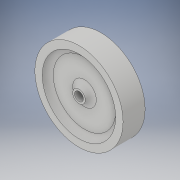
# Autodesk Inventor part: Part7
Saved by Autodesk Inventor 2018 (Build 220112000, 112)
## iProperties
Created: 2018-07-02
Part Number: Part7
Material: Generic
Document SubType Name: Modeling
Designer: s-2512711
Density: 1 g/cm^3
Appearance: Default
Author: s-2512711
Autodesk Inventor part; units mm, degrees
ref_plane "YZ Plane" through (0, 0, 0) normal (1, 0, 0) x (0, 1, 0)
ref_plane "XZ Plane" through (0, 0, 0) normal (0, 1, 0) x (-1, 0, 0)
ref_plane "XY Plane" through (0, 0, 0) normal (0, 0, 1) x (1, 0, 0)
sketch "Sketch1" plane through (0, 0, 0) normal (0, 0, 1) x (1, 0, 0)
  circle A0 centre (0, 0) radius 7.6581
  circle A1 centre (0, 0) radius 10.1981
  circle A2 centre (0, 0) radius 76.2
  circle A3 centre (0, 0) radius 63.5
  dimension "d0" = 15.3162
  dimension "d1" = 20.3962
  dimension "d2" = 152.4
  dimension "d3" = 127
  constraints: 4 centre point, 4 coincident
  measures "d0" diameter of A0
  measures "d1" diameter of A1
  measures "d2" diameter of A2
  measures "d3" diameter of A3
extrude "Extrusion1" add sketch "Sketch1" along normal blind 38.1
sketch "Sketch2" plane through (0, 0, 38.1) normal (0, 0, 1) x (1, 0, 0)
  circle A0 centre (0, 0) radius 10.1981
  circle A1 centre (0, 0) radius 63.5
  constraints: 2 centre point, 2 coincident
extrude "Extrusion2" add sketch "Sketch2" against normal blind 28.575
sketch "Sketch3" plane through (0, 0, 38.1) normal (0, 0, 1) x (1, 0, 0)
  circle A0 centre (0, 0) radius 10.8988
  circle A1 centre (0, 0) radius 63.5
  constraints: 2 centre point, 2 coincident
extrude "Extrusion3" cut sketch "Sketch3" against normal blind 9.525
fillet "Fillet1" radius 9.525 2 edges at (-10.1981, 0, 9.525) (-63.5, 0, 9.525)
fillet "Fillet2" radius 9.525 2 edges at (-63.5, 0, 28.575) (-10.8988, 0, 28.575)
sketch "Sketch4" plane through (0, 0, 0) normal (0, 0, -1) x (-1, 0, 0)
  line L0 (-9.1597, 73.9585) -> (12.5018, 73.9585) construction
  line L1 (12.5018, 73.9585) -> (12.5018, 68.6979) construction
  line L2 (12.5018, 68.6979) -> (-9.1597, 68.6979) construction
  line L3 (-9.1597, 68.6979) -> (-9.1597, 73.9585) construction
  spline S0 degree 2 poles (-6.9244, 72.9038) (-6.9244, 72.7062) (-7.0651, 72.3506) (-7.1911, 72.227) knots 0 0 0 1 2 2 2
  spline S1 degree 2 poles (-7.1911, 72.227) (-7.3492, 72.0714) (-7.7765, 71.9109) (-8.1026, 71.9109) knots 0 0 0 1 2 2 2
  line L4 (-8.1026, 71.9109) -> (-8.4459, 71.9109)
  line L5 (-8.4459, 71.9109) -> (-8.4459, 70.7747)
  line L6 (-8.4459, 70.7747) -> (-8.851, 70.7747)
  line L7 (-8.851, 70.7747) -> (-8.851, 73.8227)
  line L8 (-8.851, 73.8227) -> (-8.0853, 73.8227)
  spline S2 degree 2 poles (-8.0853, 73.8227) (-7.8136, 73.8227) (-7.4332, 73.7338) (-7.2874, 73.6325) knots 0 0 0 1 2 2 2
  spline S3 degree 2 poles (-7.2874, 73.6325) (-7.117, 73.5164) (-6.9244, 73.1582) (-6.9244, 72.9038) knots 0 0 0 1 2 2 2
  spline S4 degree 2 poles (-7.3467, 72.8915) (-7.3467, 73.0496) (-7.4554, 73.2817) (-7.5666, 73.3558) knots 0 0 0 1 2 2 2
  spline S5 degree 2 poles (-7.5666, 73.3558) (-7.6629, 73.4201) (-7.9198, 73.4719) (-8.11, 73.4719) knots 0 0 0 1 2 2 2
  line L9 (-8.11, 73.4719) -> (-8.4459, 73.4719)
  line L10 (-8.4459, 73.4719) -> (-8.4459, 72.2567)
  line L11 (-8.4459, 72.2567) -> (-8.1692, 72.2567)
  spline S6 degree 2 poles (-8.1692, 72.2567) (-7.9222, 72.2567) (-7.6184, 72.3357) (-7.5196, 72.4395) knots 0 0 0 1 2 2 2
  spline S7 degree 2 poles (-7.5196, 72.4395) (-7.4282, 72.5309) (-7.3467, 72.7458) (-7.3467, 72.8915) knots 0 0 0 1 2 2 2
  line L12 (-5.3559, 72.6494) -> (-5.3757, 72.6494)
  spline S8 degree 2 poles (-5.3757, 72.6494) (-5.4201, 72.6618) (-5.5164, 72.6667) (-5.5831, 72.6667) knots 0 0 0 1 2 2 2
  spline S9 degree 2 poles (-5.5831, 72.6667) (-5.7387, 72.6667) (-6.045, 72.5309) (-6.1833, 72.3975) knots 0 0 0 1 2 2 2
  line L13 (-6.1833, 72.3975) -> (-6.1833, 70.7747)
  line L14 (-6.1833, 70.7747) -> (-6.5687, 70.7747)
  line L15 (-6.5687, 70.7747) -> (-6.5687, 73.0619)
  line L16 (-6.5687, 73.0619) -> (-6.1833, 73.0619)
  line L17 (-6.1833, 73.0619) -> (-6.1833, 72.7211)
  spline S10 degree 2 poles (-6.1833, 72.7211) (-5.9734, 72.9088) (-5.6597, 73.0619) (-5.5115, 73.0619) knots 0 0 0 1 2 2 2
  spline S11 degree 2 poles (-5.5115, 73.0619) (-5.4522, 73.0619) (-5.3929, 73.057) (-5.3559, 73.0496) knots 0 0 0 1 2 2 2
  line L18 (-5.3559, 73.0496) -> (-5.3559, 72.6494)
  spline S12 degree 2 poles (-4.0641, 70.7228) (-4.6124, 70.7228) (-5.2151, 71.3378) (-5.2151, 71.9059) knots 0 0 0 1 2 2 2
  spline S13 degree 2 poles (-5.2151, 71.9059) (-5.2151, 72.4642) (-4.6297, 73.1261) (-4.1579, 73.1261) knots 0 0 0 1 2 2 2
  spline S14 degree 2 poles (-4.1579, 73.1261) (-3.9455, 73.1261) (-3.617, 73.0026) (-3.496, 72.8717) knots 0 0 0 1 2 2 2
  spline S15 degree 2 poles (-3.496, 72.8717) (-3.3725, 72.7408) (-3.2416, 72.3629) (-3.2416, 72.0887) knots 0 0 0 1 2 2 2
  line L19 (-3.2416, 72.0887) -> (-3.2416, 71.8788)
  line L20 (-3.2416, 71.8788) -> (-4.8248, 71.8788)
  spline S16 degree 2 poles (-4.8248, 71.8788) (-4.8248, 71.4811) (-4.4247, 71.0587) (-4.069, 71.0587) knots 0 0 0 1 2 2 2
  spline S17 degree 2 poles (-4.069, 71.0587) (-3.943, 71.0587) (-3.6985, 71.1155) (-3.5997, 71.16) knots 0 0 0 1 2 2 2
  spline S18 degree 2 poles (-3.5997, 71.16) (-3.496, 71.2094) (-3.3527, 71.2959) (-3.3058, 71.3354) knots 0 0 0 1 2 2 2
  line L21 (-3.3058, 71.3354) -> (-3.2835, 71.3354)
  line L22 (-3.2835, 71.3354) -> (-3.2835, 70.9155)
  spline S19 degree 2 poles (-3.2835, 70.9155) (-3.3502, 70.8883) (-3.5528, 70.8093) (-3.6318, 70.787) knots 0 0 0 1 2 2 2
  spline S20 degree 2 poles (-3.6318, 70.787) (-3.743, 70.7549) (-3.9258, 70.7228) (-4.0641, 70.7228) knots 0 0 0 1 2 2 2
  spline S21 degree 2 poles (-3.617, 72.1727) (-3.6219, 72.3283) (-3.6862, 72.5556) (-3.7479, 72.6321) knots 0 0 0 1 2 2 2
  spline S22 degree 2 poles (-3.7479, 72.6321) (-3.8146, 72.7186) (-4.0246, 72.81) (-4.1802, 72.81) knots 0 0 0 1 2 2 2
  spline S23 degree 2 poles (-4.1802, 72.81) (-4.3333, 72.81) (-4.5482, 72.7186) (-4.6371, 72.6297) knots 0 0 0 1 2 2 2
  spline S24 degree 2 poles (-4.6371, 72.6297) (-4.7236, 72.5383) (-4.8125, 72.3184) (-4.8248, 72.1727) knots 0 0 0 1 2 2 2
  line L23 (-4.8248, 72.1727) -> (-3.617, 72.1727)
  spline S25 degree 2 poles (-2.1597, 70.7302) (-2.4734, 70.7302) (-2.8266, 71.0884) (-2.8266, 71.4762) knots 0 0 0 1 2 2 2
  line L24 (-2.8266, 71.4762) -> (-2.8266, 72.7433)
  line L25 (-2.8266, 72.7433) -> (-3.0859, 72.7433)
  line L26 (-3.0859, 72.7433) -> (-3.0859, 73.0619)
  line L27 (-3.0859, 73.0619) -> (-2.8266, 73.0619)
  line L28 (-2.8266, 73.0619) -> (-2.8266, 73.7189)
  line L29 (-2.8266, 73.7189) -> (-2.4413, 73.7189)
  line L30 (-2.4413, 73.7189) -> (-2.4413, 73.0619)
  line L31 (-2.4413, 73.0619) -> (-1.7324, 73.0619)
  line L32 (-1.7324, 73.0619) -> (-1.7324, 72.7433)
  line L33 (-1.7324, 72.7433) -> (-2.4413, 72.7433)
  line L34 (-2.4413, 72.7433) -> (-2.4413, 71.654)
  spline S26 degree 2 poles (-2.4413, 71.654) (-2.4413, 71.4811) (-2.4289, 71.2909) (-2.3869, 71.2094) knots 0 0 0 1 2 2 2
  spline S27 degree 2 poles (-2.3869, 71.2094) (-2.3524, 71.1378) (-2.1967, 71.0661) (-2.0634, 71.0661) knots 0 0 0 1 2 2 2
  spline S28 degree 2 poles (-2.0634, 71.0661) (-1.9695, 71.0661) (-1.7941, 71.123) (-1.7546, 71.1402) knots 0 0 0 1 2 2 2
  line L35 (-1.7546, 71.1402) -> (-1.7324, 71.1402)
  line L36 (-1.7324, 71.1402) -> (-1.7324, 70.7944)
  spline S29 degree 2 poles (-1.7324, 70.7944) (-1.8411, 70.7648) (-2.0634, 70.7302) (-2.1597, 70.7302) knots 0 0 0 1 2 2 2
  spline S30 degree 2 poles (-0.4554, 70.7228) (-1.0037, 70.7228) (-1.6064, 71.3378) (-1.6064, 71.9059) knots 0 0 0 1 2 2 2
  spline S31 degree 2 poles (-1.6064, 71.9059) (-1.6064, 72.4642) (-1.021, 73.1261) (-0.5492, 73.1261) knots 0 0 0 1 2 2 2
  spline S32 degree 2 poles (-0.5492, 73.1261) (-0.3368, 73.1261) (-0.0083, 73.0026) (0.1127, 72.8717) knots 0 0 0 1 2 2 2
  spline S33 degree 2 poles (0.1127, 72.8717) (0.2362, 72.7408) (0.3671, 72.3629) (0.3671, 72.0887) knots 0 0 0 1 2 2 2
  line L37 (0.3671, 72.0887) -> (0.3671, 71.8788)
  line L38 (0.3671, 71.8788) -> (-1.2161, 71.8788)
  spline S34 degree 2 poles (-1.2161, 71.8788) (-1.2161, 71.4811) (-0.816, 71.0587) (-0.4603, 71.0587) knots 0 0 0 1 2 2 2
  spline S35 degree 2 poles (-0.4603, 71.0587) (-0.3344, 71.0587) (-0.0898, 71.1155) (0.009, 71.16) knots 0 0 0 1 2 2 2
  spline S36 degree 2 poles (0.009, 71.16) (0.1127, 71.2094) (0.256, 71.2959) (0.3029, 71.3354) knots 0 0 0 1 2 2 2
  line L39 (0.3029, 71.3354) -> (0.3251, 71.3354)
  line L40 (0.3251, 71.3354) -> (0.3251, 70.9155)
  spline S37 degree 2 poles (0.3251, 70.9155) (0.2585, 70.8883) (0.0559, 70.8093) (-0.0231, 70.787) knots 0 0 0 1 2 2 2
  spline S38 degree 2 poles (-0.0231, 70.787) (-0.1343, 70.7549) (-0.3171, 70.7228) (-0.4554, 70.7228) knots 0 0 0 1 2 2 2
  spline S39 degree 2 poles (-0.0083, 72.1727) (-0.0132, 72.3283) (-0.0775, 72.5556) (-0.1392, 72.6321) knots 0 0 0 1 2 2 2
  spline S40 degree 2 poles (-0.1392, 72.6321) (-0.2059, 72.7186) (-0.4159, 72.81) (-0.5715, 72.81) knots 0 0 0 1 2 2 2
  spline S41 degree 2 poles (-0.5715, 72.81) (-0.7246, 72.81) (-0.9395, 72.7186) (-1.0284, 72.6297) knots 0 0 0 1 2 2 2
  spline S42 degree 2 poles (-1.0284, 72.6297) (-1.1149, 72.5383) (-1.2038, 72.3184) (-1.2161, 72.1727) knots 0 0 0 1 2 2 2
  line L41 (-1.2161, 72.1727) -> (-0.0083, 72.1727)
  line L42 (2.5531, 70.7747) -> (2.1678, 70.7747)
  line L43 (2.1678, 70.7747) -> (2.1678, 72.0788)
  spline S43 degree 2 poles (2.1678, 72.0788) (2.1678, 72.2369) (2.1381, 72.5086) (2.0937, 72.5901) knots 0 0 0 1 2 2 2
  spline S44 degree 2 poles (2.0937, 72.5901) (2.0467, 72.6766) (1.8788, 72.7606) (1.7355, 72.7606) knots 0 0 0 1 2 2 2
  spline S45 degree 2 poles (1.7355, 72.7606) (1.5923, 72.7606) (1.2885, 72.6074) (1.1427, 72.4839) knots 0 0 0 1 2 2 2
  line L44 (1.1427, 72.4839) -> (1.1427, 70.7747)
  line L45 (1.1427, 70.7747) -> (0.7574, 70.7747)
  line L46 (0.7574, 70.7747) -> (0.7574, 73.0619)
  line L47 (0.7574, 73.0619) -> (1.1427, 73.0619)
  line L48 (1.1427, 73.0619) -> (1.1427, 72.8075)
  spline S46 degree 2 poles (1.1427, 72.8075) (1.3156, 72.9631) (1.6491, 73.1261) (1.8368, 73.1261) knots 0 0 0 1 2 2 2
  spline S47 degree 2 poles (1.8368, 73.1261) (2.1727, 73.1261) (2.5531, 72.6815) (2.5531, 72.2592) knots 0 0 0 1 2 2 2
  line L49 (2.5531, 72.2592) -> (2.5531, 70.7747)
  line L50 (4.8527, 70.7747) -> (4.4674, 70.7747)
  line L51 (4.4674, 70.7747) -> (4.4674, 71.0069)
  spline S48 degree 2 poles (4.4674, 71.0069) (4.3784, 70.9328) (4.2475, 70.834) (4.1586, 70.792) knots 0 0 0 1 2 2 2
  spline S49 degree 2 poles (4.1586, 70.792) (4.0771, 70.7525) (3.9017, 70.7105) (3.7856, 70.7105) knots 0 0 0 1 2 2 2
  spline S50 degree 2 poles (3.7856, 70.7105) (3.5979, 70.7105) (3.2818, 70.8661) (3.1706, 71.0167) knots 0 0 0 1 2 2 2
  spline S51 degree 2 poles (3.1706, 71.0167) (3.0595, 71.1674) (2.936, 71.612) (2.936, 71.901) knots 0 0 0 1 2 2 2
  spline S52 degree 2 poles (2.936, 71.901) (2.936, 72.2023) (3.0916, 72.642) (3.2274, 72.8075) knots 0 0 0 1 2 2 2
  spline S53 degree 2 poles (3.2274, 72.8075) (3.3534, 72.9557) (3.7066, 73.1261) (3.9017, 73.1261) knots 0 0 0 1 2 2 2
  spline S54 degree 2 poles (3.9017, 73.1261) (4.0722, 73.1261) (4.3266, 73.0496) (4.4674, 72.9705) knots 0 0 0 1 2 2 2
  line L52 (4.4674, 72.9705) -> (4.4674, 73.9585)
  line L53 (4.4674, 73.9585) -> (4.8527, 73.9585)
  line L54 (4.8527, 73.9585) -> (4.8527, 70.7747)
  line L55 (4.4674, 71.3304) -> (4.4674, 72.6519)
  spline S55 degree 2 poles (4.4674, 72.6519) (4.3241, 72.7211) (4.0969, 72.7729) (3.9659, 72.7729) knots 0 0 0 1 2 2 2
  spline S56 degree 2 poles (3.9659, 72.7729) (3.6695, 72.7729) (3.3336, 72.3283) (3.3336, 71.9084) knots 0 0 0 1 2 2 2
  spline S57 degree 2 poles (3.3336, 71.9084) (3.3336, 71.5033) (3.5905, 71.076) (3.8746, 71.076) knots 0 0 0 1 2 2 2
  spline S58 degree 2 poles (3.8746, 71.076) (4.0252, 71.076) (4.3315, 71.2143) (4.4674, 71.3304) knots 0 0 0 1 2 2 2
  spline S59 degree 2 poles (7.4116, 70.7302) (7.0979, 70.7302) (6.7447, 71.0884) (6.7447, 71.4762) knots 0 0 0 1 2 2 2
  line L56 (6.7447, 71.4762) -> (6.7447, 72.7433)
  line L57 (6.7447, 72.7433) -> (6.4854, 72.7433)
  line L58 (6.4854, 72.7433) -> (6.4854, 73.0619)
  line L59 (6.4854, 73.0619) -> (6.7447, 73.0619)
  line L60 (6.7447, 73.0619) -> (6.7447, 73.7189)
  line L61 (6.7447, 73.7189) -> (7.13, 73.7189)
  line L62 (7.13, 73.7189) -> (7.13, 73.0619)
  line L63 (7.13, 73.0619) -> (7.8389, 73.0619)
  line L64 (7.8389, 73.0619) -> (7.8389, 72.7433)
  line L65 (7.8389, 72.7433) -> (7.13, 72.7433)
  line L66 (7.13, 72.7433) -> (7.13, 71.654)
  spline S60 degree 2 poles (7.13, 71.654) (7.13, 71.4811) (7.1424, 71.2909) (7.1844, 71.2094) knots 0 0 0 1 2 2 2
  spline S61 degree 2 poles (7.1844, 71.2094) (7.219, 71.1378) (7.3746, 71.0661) (7.508, 71.0661) knots 0 0 0 1 2 2 2
  spline S62 degree 2 poles (7.508, 71.0661) (7.6018, 71.0661) (7.7772, 71.123) (7.8167, 71.1402) knots 0 0 0 1 2 2 2
  line L67 (7.8167, 71.1402) -> (7.8389, 71.1402)
  line L68 (7.8389, 71.1402) -> (7.8389, 70.7944)
  spline S63 degree 2 poles (7.8389, 70.7944) (7.7303, 70.7648) (7.508, 70.7302) (7.4116, 70.7302) knots 0 0 0 1 2 2 2
  line L69 (9.9187, 70.7747) -> (9.5334, 70.7747)
  line L70 (9.5334, 70.7747) -> (9.5334, 72.0788)
  spline S64 degree 2 poles (9.5334, 72.0788) (9.5334, 72.2369) (9.5037, 72.5086) (9.4593, 72.5901) knots 0 0 0 1 2 2 2
  spline S65 degree 2 poles (9.4593, 72.5901) (9.4123, 72.6766) (9.2444, 72.7606) (9.1011, 72.7606) knots 0 0 0 1 2 2 2
  spline S66 degree 2 poles (9.1011, 72.7606) (8.9579, 72.7606) (8.654, 72.6074) (8.5083, 72.4839) knots 0 0 0 1 2 2 2
  line L71 (8.5083, 72.4839) -> (8.5083, 70.7747)
  line L72 (8.5083, 70.7747) -> (8.123, 70.7747)
  line L73 (8.123, 70.7747) -> (8.123, 73.9585)
  line L74 (8.123, 73.9585) -> (8.5083, 73.9585)
  line L75 (8.5083, 73.9585) -> (8.5083, 72.8075)
  spline S67 degree 2 poles (8.5083, 72.8075) (8.6812, 72.9631) (9.0147, 73.1261) (9.2024, 73.1261) knots 0 0 0 1 2 2 2
  spline S68 degree 2 poles (9.2024, 73.1261) (9.5383, 73.1261) (9.9187, 72.6815) (9.9187, 72.2592) knots 0 0 0 1 2 2 2
  line L76 (9.9187, 72.2592) -> (9.9187, 70.7747)
  line L77 (10.8524, 70.7747) -> (10.467, 70.7747)
  line L78 (10.467, 70.7747) -> (10.467, 73.0619)
  line L79 (10.467, 73.0619) -> (10.8524, 73.0619)
  line L80 (10.8524, 73.0619) -> (10.8524, 70.7747)
  line L81 (10.8795, 73.4423) -> (10.4423, 73.4423)
  line L82 (10.4423, 73.4423) -> (10.4423, 73.8424)
  line L83 (10.4423, 73.8424) -> (10.8795, 73.8424)
  line L84 (10.8795, 73.8424) -> (10.8795, 73.4423)
  spline S69 degree 2 poles (12.0355, 70.7203) (11.8058, 70.7203) (11.4081, 70.8438) (11.2772, 70.913) knots 0 0 0 1 2 2 2
  line L85 (11.2772, 70.913) -> (11.2772, 71.3453)
  line L86 (11.2772, 71.3453) -> (11.297, 71.3453)
  spline S70 degree 2 poles (11.297, 71.3453) (11.3464, 71.3057) (11.4797, 71.2119) (11.5909, 71.16) knots 0 0 0 1 2 2 2
  spline S71 degree 2 poles (11.5909, 71.16) (11.6872, 71.1131) (11.9243, 71.0439) (12.0503, 71.0439) knots 0 0 0 1 2 2 2
  spline S72 degree 2 poles (12.0503, 71.0439) (12.1417, 71.0439) (12.3517, 71.0859) (12.4011, 71.1205) knots 0 0 0 1 2 2 2
  spline S73 degree 2 poles (12.4011, 71.1205) (12.4727, 71.1674) (12.5369, 71.2736) (12.5369, 71.3823) knots 0 0 0 1 2 2 2
  spline S74 degree 2 poles (12.5369, 71.3823) (12.5369, 71.5182) (12.3887, 71.6589) (12.1985, 71.7059) knots 0 0 0 1 2 2 2
  spline S75 degree 2 poles (12.1985, 71.7059) (12.1244, 71.7232) (11.8873, 71.7726) (11.786, 71.7997) knots 0 0 0 1 2 2 2
  spline S76 degree 2 poles (11.786, 71.7997) (11.5242, 71.8763) (11.2871, 72.1925) (11.2871, 72.4172) knots 0 0 0 1 2 2 2
  spline S77 degree 2 poles (11.2871, 72.4172) (11.2871, 72.7285) (11.7539, 73.1163) (12.1392, 73.1163) knots 0 0 0 1 2 2 2
  spline S78 degree 2 poles (12.1392, 73.1163) (12.3294, 73.1163) (12.7147, 73.0224) (12.8457, 72.9508) knots 0 0 0 1 2 2 2
  line L87 (12.8457, 72.9508) -> (12.8457, 72.5383)
  line L88 (12.8457, 72.5383) -> (12.8259, 72.5383)
  spline S79 degree 2 poles (12.8259, 72.5383) (12.6777, 72.6568) (12.3171, 72.7927) (12.1318, 72.7927) knots 0 0 0 1 2 2 2
  spline S80 degree 2 poles (12.1318, 72.7927) (11.9416, 72.7927) (11.6798, 72.6321) (11.6798, 72.4716) knots 0 0 0 1 2 2 2
  spline S81 degree 2 poles (11.6798, 72.4716) (11.6798, 72.3259) (11.8354, 72.1851) (12.0083, 72.1406) knots 0 0 0 1 2 2 2
  spline S82 degree 2 poles (12.0083, 72.1406) (12.0923, 72.1184) (12.3047, 72.0739) (12.4208, 72.0467) knots 0 0 0 1 2 2 2
  spline S83 degree 2 poles (12.4208, 72.0467) (12.6728, 71.9825) (12.9296, 71.6886) (12.9296, 71.4342) knots 0 0 0 1 2 2 2
  spline S84 degree 2 poles (12.9296, 71.4342) (12.9296, 71.286) (12.8135, 71.0242) (12.6999, 70.9278) knots 0 0 0 1 2 2 2
  spline S85 degree 2 poles (12.6999, 70.9278) (12.5789, 70.8266) (12.2701, 70.7203) (12.0355, 70.7203) knots 0 0 0 1 2 2 2
  line L89 (-8.4879, 65.7562) -> (-8.8732, 65.7562)
  line L90 (-8.8732, 65.7562) -> (-8.8732, 68.0435)
  line L91 (-8.8732, 68.0435) -> (-8.4879, 68.0435)
  line L92 (-8.4879, 68.0435) -> (-8.4879, 65.7562)
  line L93 (-8.4607, 68.4238) -> (-8.8979, 68.4238)
  line L94 (-8.8979, 68.4238) -> (-8.8979, 68.824)
  line L95 (-8.8979, 68.824) -> (-8.4607, 68.824)
  line L96 (-8.4607, 68.824) -> (-8.4607, 68.4238)
  spline S86 degree 2 poles (-7.3047, 65.7019) (-7.5344, 65.7019) (-7.9321, 65.8254) (-8.063, 65.8945) knots 0 0 0 1 2 2 2
  line L97 (-8.063, 65.8945) -> (-8.063, 66.3268)
  line L98 (-8.063, 66.3268) -> (-8.0433, 66.3268)
  spline S87 degree 2 poles (-8.0433, 66.3268) (-7.9939, 66.2873) (-7.8605, 66.1934) (-7.7493, 66.1416) knots 0 0 0 1 2 2 2
  spline S88 degree 2 poles (-7.7493, 66.1416) (-7.653, 66.0946) (-7.4159, 66.0255) (-7.2899, 66.0255) knots 0 0 0 1 2 2 2
  spline S89 degree 2 poles (-7.2899, 66.0255) (-7.1985, 66.0255) (-6.9886, 66.0675) (-6.9392, 66.102) knots 0 0 0 1 2 2 2
  spline S90 degree 2 poles (-6.9392, 66.102) (-6.8675, 66.149) (-6.8033, 66.2552) (-6.8033, 66.3639) knots 0 0 0 1 2 2 2
  spline S91 degree 2 poles (-6.8033, 66.3639) (-6.8033, 66.4997) (-6.9515, 66.6405) (-7.1417, 66.6874) knots 0 0 0 1 2 2 2
  spline S92 degree 2 poles (-7.1417, 66.6874) (-7.2158, 66.7047) (-7.4529, 66.7541) (-7.5542, 66.7813) knots 0 0 0 1 2 2 2
  spline S93 degree 2 poles (-7.5542, 66.7813) (-7.816, 66.8579) (-8.0532, 67.174) (-8.0532, 67.3988) knots 0 0 0 1 2 2 2
  spline S94 degree 2 poles (-8.0532, 67.3988) (-8.0532, 67.71) (-7.5863, 68.0978) (-7.201, 68.0978) knots 0 0 0 1 2 2 2
  spline S95 degree 2 poles (-7.201, 68.0978) (-7.0108, 68.0978) (-6.6255, 68.0039) (-6.4946, 67.9323) knots 0 0 0 1 2 2 2
  line L99 (-6.4946, 67.9323) -> (-6.4946, 67.5198)
  line L100 (-6.4946, 67.5198) -> (-6.5143, 67.5198)
  spline S96 degree 2 poles (-6.5143, 67.5198) (-6.6625, 67.6384) (-7.0232, 67.7742) (-7.2084, 67.7742) knots 0 0 0 1 2 2 2
  spline S97 degree 2 poles (-7.2084, 67.7742) (-7.3986, 67.7742) (-7.6604, 67.6137) (-7.6604, 67.4531) knots 0 0 0 1 2 2 2
  spline S98 degree 2 poles (-7.6604, 67.4531) (-7.6604, 67.3074) (-7.5048, 67.1666) (-7.3319, 67.1221) knots 0 0 0 1 2 2 2
  spline S99 degree 2 poles (-7.3319, 67.1221) (-7.2479, 67.0999) (-7.0355, 67.0555) (-6.9194, 67.0283) knots 0 0 0 1 2 2 2
  spline S100 degree 2 poles (-6.9194, 67.0283) (-6.6675, 66.9641) (-6.4106, 66.6701) (-6.4106, 66.4157) knots 0 0 0 1 2 2 2
  spline S101 degree 2 poles (-6.4106, 66.4157) (-6.4106, 66.2675) (-6.5267, 66.0057) (-6.6403, 65.9094) knots 0 0 0 1 2 2 2
  spline S102 degree 2 poles (-6.6403, 65.9094) (-6.7613, 65.8081) (-7.0701, 65.7019) (-7.3047, 65.7019) knots 0 0 0 1 2 2 2
  spline S103 degree 2 poles (-3.8344, 65.7044) (-4.0715, 65.7044) (-4.4642, 65.8501) (-4.605, 65.9983) knots 0 0 0 1 2 2 2
  spline S104 degree 2 poles (-4.605, 65.9983) (-4.7458, 66.144) (-4.9014, 66.5936) (-4.9014, 66.8949) knots 0 0 0 1 2 2 2
  spline S105 degree 2 poles (-4.9014, 66.8949) (-4.9014, 67.1962) (-4.7409, 67.6359) (-4.605, 67.7841) knots 0 0 0 1 2 2 2
  spline S106 degree 2 poles (-4.605, 67.7841) (-4.4692, 67.9348) (-4.0665, 68.0953) (-3.8344, 68.0953) knots 0 0 0 1 2 2 2
  spline S107 degree 2 poles (-3.8344, 68.0953) (-3.6466, 68.0953) (-3.2959, 67.9891) (-3.16, 67.92) knots 0 0 0 1 2 2 2
  line L101 (-3.16, 67.92) -> (-3.16, 67.4877)
  line L102 (-3.16, 67.4877) -> (-3.1823, 67.4877)
  spline S108 degree 2 poles (-3.1823, 67.4877) (-3.2243, 67.5223) (-3.3527, 67.6112) (-3.4441, 67.6581) knots 0 0 0 1 2 2 2
  spline S109 degree 2 poles (-3.4441, 67.6581) (-3.5256, 67.6977) (-3.743, 67.7594) (-3.8418, 67.7594) knots 0 0 0 1 2 2 2
  spline S110 degree 2 poles (-3.8418, 67.7594) (-4.1406, 67.7594) (-4.5037, 67.3074) (-4.5037, 66.8949) knots 0 0 0 1 2 2 2
  spline S111 degree 2 poles (-4.5037, 66.8949) (-4.5037, 66.4923) (-4.153, 66.0403) (-3.8418, 66.0403) knots 0 0 0 1 2 2 2
  spline S112 degree 2 poles (-3.8418, 66.0403) (-3.6541, 66.0403) (-3.3132, 66.1959) (-3.1823, 66.3169) knots 0 0 0 1 2 2 2
  line L103 (-3.1823, 66.3169) -> (-3.16, 66.3169)
  line L104 (-3.16, 66.3169) -> (-3.16, 65.8847)
  spline S113 degree 2 poles (-3.16, 65.8847) (-3.2169, 65.8575) (-3.3898, 65.7809) (-3.4589, 65.7636) knots 0 0 0 1 2 2 2
  spline S114 degree 2 poles (-3.4589, 65.7636) (-3.5577, 65.734) (-3.7133, 65.7044) (-3.8344, 65.7044) knots 0 0 0 1 2 2 2
  spline S115 degree 2 poles (-0.9296, 66.8998) (-0.9296, 66.3219) (-1.4854, 65.692) (-1.9497, 65.692) knots 0 0 0 1 2 2 2
  spline S116 degree 2 poles (-1.9497, 65.692) (-2.4265, 65.692) (-2.9723, 66.3416) (-2.9723, 66.8998) knots 0 0 0 1 2 2 2
  spline S117 degree 2 poles (-2.9723, 66.8998) (-2.9723, 67.4729) (-2.4092, 68.1077) (-1.9497, 68.1077) knots 0 0 0 1 2 2 2
  spline S118 degree 2 poles (-1.9497, 68.1077) (-1.4854, 68.1077) (-0.9296, 67.4754) (-0.9296, 66.8998) knots 0 0 0 1 2 2 2
  spline S119 degree 2 poles (-1.3273, 66.8998) (-1.3273, 67.3444) (-1.6509, 67.7767) (-1.9497, 67.7767) knots 0 0 0 1 2 2 2
  spline S120 degree 2 poles (-1.9497, 67.7767) (-2.2486, 67.7767) (-2.5747, 67.3444) (-2.5747, 66.8998) knots 0 0 0 1 2 2 2
  spline S121 degree 2 poles (-2.5747, 66.8998) (-2.5747, 66.4676) (-2.2486, 66.023) (-1.9497, 66.023) knots 0 0 0 1 2 2 2
  spline S122 degree 2 poles (-1.9497, 66.023) (-1.6533, 66.023) (-1.3273, 66.4602) (-1.3273, 66.8998) knots 0 0 0 1 2 2 2
  line L105 (-0.1417, 65.7562) -> (-0.527, 65.7562)
  line L106 (-0.527, 65.7562) -> (-0.527, 68.9401)
  line L107 (-0.527, 68.9401) -> (-0.1417, 68.9401)
  line L108 (-0.1417, 68.9401) -> (-0.1417, 65.7562)
  spline S123 degree 2 poles (1.0414, 65.7019) (0.8117, 65.7019) (0.4141, 65.8254) (0.2832, 65.8945) knots 0 0 0 1 2 2 2
  line L109 (0.2832, 65.8945) -> (0.2832, 66.3268)
  line L110 (0.2832, 66.3268) -> (0.3029, 66.3268)
  spline S124 degree 2 poles (0.3029, 66.3268) (0.3523, 66.2873) (0.4857, 66.1934) (0.5968, 66.1416) knots 0 0 0 1 2 2 2
  spline S125 degree 2 poles (0.5968, 66.1416) (0.6932, 66.0946) (0.9303, 66.0255) (1.0563, 66.0255) knots 0 0 0 1 2 2 2
  spline S126 degree 2 poles (1.0563, 66.0255) (1.1477, 66.0255) (1.3576, 66.0675) (1.407, 66.102) knots 0 0 0 1 2 2 2
  spline S127 degree 2 poles (1.407, 66.102) (1.4786, 66.149) (1.5429, 66.2552) (1.5429, 66.3639) knots 0 0 0 1 2 2 2
  spline S128 degree 2 poles (1.5429, 66.3639) (1.5429, 66.4997) (1.3947, 66.6405) (1.2045, 66.6874) knots 0 0 0 1 2 2 2
  spline S129 degree 2 poles (1.2045, 66.6874) (1.1304, 66.7047) (0.8932, 66.7541) (0.792, 66.7813) knots 0 0 0 1 2 2 2
  spline S130 degree 2 poles (0.792, 66.7813) (0.5302, 66.8579) (0.293, 67.174) (0.293, 67.3988) knots 0 0 0 1 2 2 2
  spline S131 degree 2 poles (0.293, 67.3988) (0.293, 67.71) (0.7599, 68.0978) (1.1452, 68.0978) knots 0 0 0 1 2 2 2
  spline S132 degree 2 poles (1.1452, 68.0978) (1.3354, 68.0978) (1.7207, 68.0039) (1.8516, 67.9323) knots 0 0 0 1 2 2 2
  line L111 (1.8516, 67.9323) -> (1.8516, 67.5198)
  line L112 (1.8516, 67.5198) -> (1.8319, 67.5198)
  spline S133 degree 2 poles (1.8319, 67.5198) (1.6837, 67.6384) (1.323, 67.7742) (1.1378, 67.7742) knots 0 0 0 1 2 2 2
  spline S134 degree 2 poles (1.1378, 67.7742) (0.9476, 67.7742) (0.6858, 67.6137) (0.6858, 67.4531) knots 0 0 0 1 2 2 2
  spline S135 degree 2 poles (0.6858, 67.4531) (0.6858, 67.3074) (0.8414, 67.1666) (1.0143, 67.1221) knots 0 0 0 1 2 2 2
  spline S136 degree 2 poles (1.0143, 67.1221) (1.0983, 67.0999) (1.3107, 67.0555) (1.4268, 67.0283) knots 0 0 0 1 2 2 2
  spline S137 degree 2 poles (1.4268, 67.0283) (1.6787, 66.9641) (1.9356, 66.6701) (1.9356, 66.4157) knots 0 0 0 1 2 2 2
  spline S138 degree 2 poles (1.9356, 66.4157) (1.9356, 66.2675) (1.8195, 66.0057) (1.7059, 65.9094) knots 0 0 0 1 2 2 2
  spline S139 degree 2 poles (1.7059, 65.9094) (1.5849, 65.8081) (1.2761, 65.7019) (1.0414, 65.7019) knots 0 0 0 1 2 2 2
  spline S140 degree 2 poles (4.1734, 66.8998) (4.1734, 66.3219) (3.6177, 65.692) (3.1533, 65.692) knots 0 0 0 1 2 2 2
  spline S141 degree 2 poles (3.1533, 65.692) (2.6766, 65.692) (2.1307, 66.3416) (2.1307, 66.8998) knots 0 0 0 1 2 2 2
  spline S142 degree 2 poles (2.1307, 66.8998) (2.1307, 67.4729) (2.6939, 68.1077) (3.1533, 68.1077) knots 0 0 0 1 2 2 2
  spline S143 degree 2 poles (3.1533, 68.1077) (3.6177, 68.1077) (4.1734, 67.4754) (4.1734, 66.8998) knots 0 0 0 1 2 2 2
  spline S144 degree 2 poles (3.7758, 66.8998) (3.7758, 67.3444) (3.4522, 67.7767) (3.1533, 67.7767) knots 0 0 0 1 2 2 2
  spline S145 degree 2 poles (3.1533, 67.7767) (2.8544, 67.7767) (2.5284, 67.3444) (2.5284, 66.8998) knots 0 0 0 1 2 2 2
  spline S146 degree 2 poles (2.5284, 66.8998) (2.5284, 66.4676) (2.8544, 66.023) (3.1533, 66.023) knots 0 0 0 1 2 2 2
  spline S147 degree 2 poles (3.1533, 66.023) (3.4497, 66.023) (3.7758, 66.4602) (3.7758, 66.8998) knots 0 0 0 1 2 2 2
  line L113 (6.3643, 65.7562) -> (5.979, 65.7562)
  line L114 (5.979, 65.7562) -> (5.979, 67.0604)
  spline S148 degree 2 poles (5.979, 67.0604) (5.979, 67.2185) (5.9494, 67.4902) (5.9049, 67.5717) knots 0 0 0 1 2 2 2
  spline S149 degree 2 poles (5.9049, 67.5717) (5.858, 67.6581) (5.69, 67.7421) (5.5468, 67.7421) knots 0 0 0 1 2 2 2
  spline S150 degree 2 poles (5.5468, 67.7421) (5.4035, 67.7421) (5.0997, 67.589) (4.954, 67.4655) knots 0 0 0 1 2 2 2
  line L115 (4.954, 67.4655) -> (4.954, 65.7562)
  line L116 (4.954, 65.7562) -> (4.5686, 65.7562)
  line L117 (4.5686, 65.7562) -> (4.5686, 68.0435)
  line L118 (4.5686, 68.0435) -> (4.954, 68.0435)
  line L119 (4.954, 68.0435) -> (4.954, 67.7891)
  spline S151 degree 2 poles (4.954, 67.7891) (5.1269, 67.9447) (5.4603, 68.1077) (5.648, 68.1077) knots 0 0 0 1 2 2 2
  spline S152 degree 2 poles (5.648, 68.1077) (5.984, 68.1077) (6.3643, 67.6631) (6.3643, 67.2407) knots 0 0 0 1 2 2 2
  line L120 (6.3643, 67.2407) -> (6.3643, 65.7562)
  point P0 (0, 0)
  constraints: 2 other
emboss "Emboss1" sketch "Sketch4" operation cut depth 2.54 direction (0, 0, 1)
body "Solid1"
